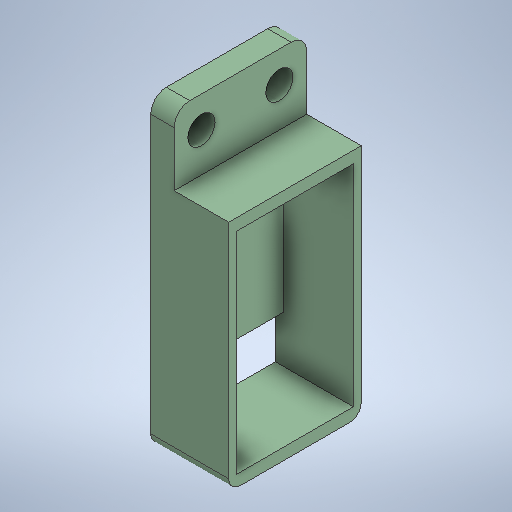
# Autodesk Inventor part: support_tof_actionneur_panneaux_solaires
Saved by Autodesk Inventor 2025 (Build 290162000, 162)
## iProperties
Created: 2024-04-13
Part Number: support_tof_actionneur_panneaux_solaires
Material: Générique
Document SubType Name: Modeling
Designer: chass
Density: 1 g/cm^3
Appearance: Par défaut
Author: chass
Autodesk Inventor part; units mm, degrees
ref_plane "YZ Plane" through (0, 0, 0) normal (1, 0, 0) x (0, 1, 0)
ref_plane "XZ Plane" through (0, 0, 0) normal (0, 1, 0) x (-1, 0, 0)
ref_plane "XY Plane" through (0, 0, 0) normal (0, 0, 1) x (1, 0, 0)
sketch "Esquisse1" plane through (0, 0, 0) normal (1, 0, 0) x (0, 1, 0)
  line L0 (15, 8.5) -> (-15, 8.5)
  line L1 (-15, 8.5) -> (-15, -8.5)
  line L2 (-15, -8.5) -> (15, -8.5)
  line L3 (15, -8.5) -> (15, 8.5)
  point P0 (0, 0)
  point P1 (0, 0)
  point P2 (0, 0)
  dimension "d4" = 30
  dimension "d5" = 17
  constraints: 8 end point, 2 parallel, 1 coincident, 1 horizontal, 1 perpendicular
  measures "d4" distance of L1.end L2.end
  measures "d5" distance of L2.end L0.start
extrude "Extrusion1" add sketch "Esquisse1" along normal blind 10
sketch "Esquisse2" plane through (10, 0, 0) normal (1, 0, 0) x (0, 0, -1)
  line L0 (-7.5, 13.5) -> (7.5, 13.5)
  line L1 (7.5, 13.5) -> (7.5, -13.5)
  line L2 (7.5, -13.5) -> (-7.5, -13.5)
  line L3 (-7.5, -13.5) -> (-7.5, 13.5)
  line L4 (-7.5, 13.5) -> (7.5, -13.5)
  line L5 (-7.5, -13.5) -> (7.5, 13.5)
  point P0 (0, 0)
  point P1 (0, 0)
  point P2 (0, 0)
  dimension "d8" = 27
  dimension "d9" = 15
  constraints: 12 end point, 2 midpoint, 2 parallel, 1 coincident, 1 horizontal, 1 perpendicular
  measures "d8" distance of L0.end L1.end
  measures "d9" distance of L0.start L0.end
extrude "Extrusion2" cut sketch "Esquisse2" against normal blind 9
sketch "Esquisse3" plane through (1, 0, 0) normal (1, 0, 0) x (0, 0, -1)
  line L0 (7.5, -13.5) -> (-7.5, -13.5) projected
  line L1 (7.5, 13.5) -> (7.5, -13.5) projected
  line L2 (-7.5, -13.5) -> (7.5, -13.5)
  line L3 (7.5, -13.5) -> (7.5, -7.5)
  line L4 (7.5, -7.5) -> (-7.5, -7.5)
  line L5 (-7.5, -7.5) -> (-7.5, -13.5)
  point P0 (0, 0)
  dimension "d12" = 6
  constraints: 8 end point, 2 parallel, 1 horizontal, 1 perpendicular, 1 point on line
  measures "d12" distance of L3.end L2.end
extrude "Extrusion3" cut sketch "Esquisse3" against normal blind 9
sketch "Esquisse4" plane through (0, 15, 8.5) normal (0, 1, 0) x (1, 0, 0)
  line L0 (0, 0) -> (0, 17) projected
  line L1 (0, 0) -> (10, 0) projected
  line L2 (0, 17) -> (3, 17)
  line L3 (3, 17) -> (3, 0)
  line L4 (3, 0) -> (0, 0)
  line L5 (0, 0) -> (0, 17)
  point P0 (0, 8.5)
  constraints: 8 end point, 2 parallel, 1 horizontal, 1 perpendicular, 1 point on line
extrude "Extrusion4" add sketch "Esquisse4" along normal blind 9
sketch "Esquisse5" plane through (3, 15, 8.5) normal (1, 0, 0) x (0, 0, -1)
  circle A0 centre (13.5, 5) radius 1.75
  line L0 (17, 9) -> (0, 9) projected
  line L1 (8.5, 9) -> (8.5, 0)
  line L2 (17, 0) -> (0, 0) projected
  circle A1 centre (3.5, 5) radius 1.75
  point P0 (8.5, -15)
  dimension "d17" = 3.5
  dimension "d18" = 5
  dimension "d19" = 4
  constraints: 2 centre point, 2 end point, 2 midpoint, 1 symmetric about line, 1 other
  measures "d17" diameter of A0
  measures "d18" distance from line of L1 A0.centre
  measures "d19" distance from line of L0 A0.centre
extrude "Extrusion5" cut sketch "Esquisse5" against normal blind 3
fillet "Congé1" radius 2 2 edges at (1.5, 24, -8.5) (1.5, 24, 8.5)
fillet "Congé2" radius 1.5 2 edges at (5, -15, 8.5) (5, -15, -8.5)
